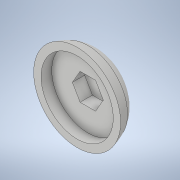
# Autodesk Inventor part: nut_cover1
Saved by Autodesk Inventor 2020 (Build 240168000, 168)
## iProperties
Created: 2018-05-22
Part Number: nut_cover1
Material: Generic
Document SubType Name: Modeling
Designer: stedrock
Density: 1 g/cm^3
Appearance: Default
Author: stedrock
Autodesk Inventor part; units mm, degrees
ref_plane "YZ Plane" through (0, 0, 0) normal (1, 0, 0) x (0, 1, 0)
ref_plane "XZ Plane" through (0, 0, 0) normal (0, 1, 0) x (-1, 0, 0)
ref_plane "XY Plane" through (0, 0, 0) normal (0, 0, 1) x (1, 0, 0)
sketch "Sketch1" plane through (0, 0, 0) normal (0, 0, 1) x (1, 0, 0)
  line L0 (0, 0) -> (26.2535, 0) construction
  line L1 (4.3301, 0) -> (2.1651, -3.75)
  line L2 (2.1651, -3.75) -> (-2.1651, -3.75)
  line L3 (-2.1651, -3.75) -> (-4.3301, 0)
  line L4 (-4.3301, 0) -> (-2.1651, 3.75)
  line L5 (-2.1651, 3.75) -> (2.1651, 3.75)
  line L6 (2.1651, 3.75) -> (4.3301, 0)
  circle A0 centre (0, 0) radius 10.1
  circle A1 centre (0, 0) radius 11.1
  dimension "d0" = 7.5
  dimension "d1" = 20.2
  dimension "d2" = 22.2
  constraints: 14 end point, 3 coincident, 2 centre point, 1 horizontal, 1 point on line, 13 other
  measures "d0" distance between parallel lines of L1 L4
  measures "d1" diameter of A0
  measures "d2" diameter of A1
sketch "Sketch3" plane through (0, 0, 0) normal (0, 1, 0) x (-1, 0, 0)
  line L0 (0, 0) -> (0, -4.2)
  line L1 (11.1, 0) -> (-11.1, 0) projected
  line L2 (0, 0) -> (-26.2535, 0) construction
  line L3 (-11.1, 0) -> (0, 0)
  line L4 (-11.1, 0) -> (-11.1, 3)
  line L5 (0, -4.2) -> (-4.3301, -4.2)
  line L6 (-4.3301, 0) -> (-2.1651, 0) projected
  line L7 (-2.1651, 0) -> (-4.3301, 0) projected
  line L8 (-4.3301, -4.2) -> (-4.3301, 0) construction
  line L9 (-11.1, 3) -> (-12.1687, 3)
  arc A0 (-11.1, 0) -> (-4.3301, -4.2) centre (-4.3301, 3.3561) ccw
  arc A1 (-12.1687, 3) -> (-11.1, 0) centre (1.0167, 6.0067) ccw
  line L10 (10.1, 0) -> (-10.1, 0) projected
  line L11 (-11.1, 0) -> (-10.1, 0)
  line L12 (-10.1, 0) -> (-10.1, 3)
  line L13 (-10.1, 3) -> (-11.1, 3)
  line L14 (-11.1, 3) -> (-11.1, 0)
  dimension "d3" = 4.2
  dimension "d4" = 3
  constraints: 21 end point, 4 horizontal, 4 point on circle, 3 parallel, 2 centre point, 2 tangent, 2 vertical, 1 collinear, 1 perpendicular, 1 other
  measures "d3" distance of L0.start L0.end
  measures "d4" distance of L3.start L4.end
revolve "Revolution1" add sketch "Sketch3" angle 360 about axis through (0, 0, 0) along (0, 0, -1)
extrude "Extrusion1" cut sketch "Sketch1" against normal blind 3.45 contours L1 L2 L3 L4 L5 L6
body "Solid1"
